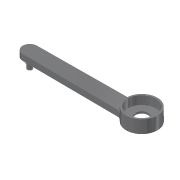
# Autodesk Inventor part: bras_moteur_1
Saved by Autodesk Inventor 2020 (Build 240168000, 168)
## iProperties
Created: 2004-05-22
Part Number: bras_moteur_1
Material: Aluminum-6061
Document SubType Name: Modélisation
Designer: françois CHAILLOT
Density: 2.71 g/cm^3
Appearance: Metal-AL-6061 (Machined)
Control State: 0
Master: False
Checked Out: False
Shininess: 66.0
Length Units: 11269
Angle Units: 11279
Time Units: 11290
Mass Units: 11283
Length Display Precision: 3
Angle Display Precision: 2
Density: 0.0
Volumn: 0.0
Area: 0.0
PropertySet Name: Model Information
Author: françois CHAILLOT
Autodesk Inventor part; units mm, degrees
ref_plane "Plan YZ" through (0, 0, 0) normal (1, 0, 0) x (0, 1, 0)
sketch "Esquisse1" plane through (0, 0, 0) normal (0, 0, 1) x (1, 0, 0)
  line L0 (-51.70019, 0) -> (420.10247, 0)
  arc A0 (0, 18) -> (0, -18) centre (0, 0) ccw
  line L1 (246.520562, 20) -> (-0.145984, 17.999408)
  line L2 (246.520562, -20) -> (-0.145984, -17.999408)
  line L3 (244.42737, 15.982892) -> (-0.113543, 13.99954)
  arc A1 (-0.113543, 13.99954) -> (-0.113537, -13.99954) centre (0, 0) ccw
  line L4 (244.427323, -15.982787) -> (-0.113537, -13.99954)
  circle A2 centre (280.0019, 0) radius 35
  circle A3 centre (280.0019, 0) radius 39
  dimension "d67" = 20
  dimension "d79" = 18
  dimension "d80" = 4
  dimension "d190" = 70
  dimension "d191" = 78
  dimension "d192" = 20
  constraints: 10 point on circle, 8 end point, 4 centre point, 4 coincident, 4 tangent, 1 point on line
  measures "d67" distance from line of L0 L2.start
  measures "d79" radius of A0
  measures "d80" distance between parallel lines of L1 L3
  measures "d190" diameter of A2
  measures "d191" diameter of A3
  measures "d192" distance from line of L0 L1.start
extrude "Extrusion7" add sketch "Esquisse1" along normal blind 15 contours A2 L0 A3 | L0 A3 A2 | A3 L3 A1 L0 A0 L1 | L2 A0 L0 A1 L4 A3
sketch "Esquisse7" plane through (0, 0, 15) normal (0, 0, 1) x (1, 0, 0)
  arc A0 (244.42737, 15.982892) -> (244.427323, -15.982787) centre (280.0019, 0) ccw
  line L0 (-0.113543, 13.99954) -> (244.42737, 15.982892)
  line L1 (244.427323, -15.982787) -> (-0.113537, -13.99954)
  arc A1 (-0.113543, 13.99954) -> (-0.113537, -13.99954) centre (0, 0) ccw
  point P0 (280, 0.667235)
extrude "Extrusion9" add sketch "Esquisse7" against normal blind 4
ref_plane "Plan de construction2" through (0, 0, 11) normal (0, 0, -1) x (-1, 0, 0)
sketch "Esquisse13" plane through (0, 0, 11) normal (0, 0, -1) x (-1, 0, 0)
  circle A0 centre (0, 0) radius 17.99
  line L0 (-65, 15) -> (-15, 15)
  line L1 (-15, 15) -> (-15, -15)
  line L2 (-15, -15) -> (-65, -15)
  line L3 (-65, -15) -> (-65, 15)
  line L4 (-65, -15) -> (-15, 15)
  line L5 (-65, -13.250714) -> (-17.915476, 15)
  line L6 (-62.084524, -15) -> (-15, 13.250714)
  line L7 (-65, 15) -> (-15, -15)
  line L8 (-62.084524, 15) -> (-15, -13.250714)
  line L9 (-65, 13.250714) -> (-17.915476, -15)
  line L10 (-137, 15.5) -> (-75, 15.5)
  line L11 (-75, 15.5) -> (-75, -15.5)
  line L12 (-75, -15.5) -> (-137, -15.5)
  line L13 (-137, -15.5) -> (-137, 15.5)
  line L14 (-137, 15.5) -> (-75, -15.5)
  line L15 (-75, 15.5) -> (-137, -15.5)
  line L16 (-133.645898, 15.5) -> (-75, -13.822949)
  line L17 (-78.354102, 15.5) -> (-137, -13.822949)
  line L18 (-75, 13.822949) -> (-133.645898, -15.5)
  line L19 (-137, 13.822949) -> (-78.354102, -15.5)
  line L20 (-75, 15.5) -> (-65, 15)
  line L21 (-65, -15) -> (-75, -15.994192)
  line L22 (-75, -15.994192) -> (-75, -15.5)
  line L23 (-195, 16) -> (-147, 16)
  line L24 (-147, 16) -> (-147, -16)
  line L25 (-147, -16) -> (-195, -16)
  line L26 (-195, -16) -> (-195, 16)
  line L27 (-195, 16) -> (-147, -16)
  line L28 (-147, 16) -> (-195, -16)
  line L29 (-192.295837, 16) -> (-147, -14.197224)
  line L30 (-195, 14.197224) -> (-149.704163, -16)
  line L31 (-149.704163, 16) -> (-195, -14.197224)
  line L32 (-147, 14.197224) -> (-192.295837, -16)
  line L33 (-238, 8) -> (-221, 10)
  line L34 (-221, 10) -> (-221, -10)
  line L35 (-221, -10) -> (-238, -8)
  line L36 (-238, 8) -> (-238, -8)
  line L37 (-217, 10.000093) -> (-205, 10.000093)
  line L38 (-205, 10.000093) -> (-205, -9.999907)
  line L39 (-205, -9.999907) -> (-217, -9.999907)
  line L40 (-217, -9.999907) -> (-217, 10.000093)
  line L41 (-195, -16) -> (-202.511566, -16.060823)
  line L42 (-195, 17.693981) -> (-195, 16)
  line L43 (-195, -16) -> (-195, -16)
  line L44 (-205, 10.000093) -> (-205, 17.174385)
  line L45 (-147, -16) -> (-137, -15.5)
  line L46 (-205, 17.174385) -> (-195, 17.693981)
  line L47 (-244.732469, -15.983444) -> (-244.732469, -15.983444)
  line L48 (-205, 10.000093) -> (-217, 10.000093)
  line L49 (-217, -9.999907) -> (-205, -9.999907)
  line L50 (-205, -9.999907) -> (-205.000086, -16.080973)
  line L51 (-205.000086, -16.080973) -> (-202.511566, -16.060823)
  line L52 (-205, 15.982892) -> (-205, -15.662243)
  line L53 (-147, 16) -> (-137, 15.5)
  arc A1 (-244.427323, -15.982787) -> (-244.42737, 15.982892) centre (-280.0019, 0) ccw
  circle A2 centre (-70, 0) radius 9
  circle A3 centre (-142, 0) radius 9
  circle A4 centre (-200, 0) radius 9
  line L54 (0, -21.588) -> (0, 28.784)
  line L55 (-244.42737, 15.982892) -> (-205, 15.982892)
  line L56 (-205, 15.982892) -> (-205, 10.000093)
  line L57 (-217, 10.000093) -> (-217, -9.999907)
  line L58 (-205, -9.999907) -> (-205, -15.662243)
  point P0 (-75, 15.186054)
  point P1 (-75, -14.19704)
  point P2 (-280, 0.667235)
  dimension "d100" = 35.98
  dimension "d104" = 50
  dimension "d109" = 1.5
  dimension "d110" = 1.5
  dimension "d118" = 1.5
  dimension "d119" = 1.5
  dimension "d128" = 31
  dimension "d131" = 1.5
  dimension "d132" = 3
  dimension "d134" = 10
  dimension "d135" = 62
  dimension "d148" = 32
  dimension "d150" = 48
  dimension "d151" = 10
  dimension "d153" = 1.5
  dimension "d154" = 3
  dimension "d155" = 1.5
  dimension "d156" = 3
  dimension "d157" = 20
  dimension "d159" = 12
  dimension "d160" = 10
  dimension "d161" = 17
  dimension "d162" = 20
  dimension "d167" = 16
  dimension "d194" = 18
  dimension "d195" = 18
  dimension "d196" = 18
  dimension "d197" = 65
  constraints: 116 end point, 25 point on line, 13 parallel, 6 perpendicular, 4 centre point, 4 coincident, 4 horizontal, 2 collinear
  measures "d100" diameter of A0
  measures "d104" distance between parallel lines of L1 L3
  measures "d109" distance between parallel lines of L6 L4
  measures "d110" distance between parallel lines of L5 L4
  measures "d118" distance between parallel lines of L8 L7
  measures "d119" distance between parallel lines of L9 L7
  measures "d128" distance between parallel lines of L12 L10
  measures "d131" distance between parallel lines of L17 L15
  measures "d132" distance between parallel lines of L18 L17
  measures "d134" distance between parallel lines of L3 L11
  measures "d135" distance between parallel lines of L13 L11
  measures "d148" distance between parallel lines of L25 L23
  measures "d150" distance between parallel lines of L24 L26
  measures "d151" distance between parallel lines of L13 L24
  measures "d153" distance between parallel lines of L29 L27
  measures "d154" distance between parallel lines of L30 L29
  measures "d155" distance between parallel lines of L31 L28
  measures "d156" distance between parallel lines of L31 L32
  measures "d157" distance between parallel lines of L39 L37
  measures "d159" distance between parallel lines of L40 L38
  measures "d160" distance between parallel lines of L26 L38
  measures "d161" distance between parallel lines of L34 L36
  measures "d162" distance of L34.end L33.end
  measures "d167" distance of L35.end L33.start
  measures "d194" diameter of A2
  measures "d195" diameter of A3
  measures "d196" diameter of A4
  measures "d197" distance between parallel lines of L54 L3
extrude "Extrusion19" add sketch "Esquisse13" along normal blind 11 contours A0 L54 | L54 A0 L1 | L1 A0 | L6 L8 L4 L1 | L1 L7 L6 L8 | L4 L8 L5 L0 | L6 L7 L4 L8 | L2 L9 L6 L7 | L4 L7 L5 L8 | L6 L9 L4 L7 | L8 L5 L7 L0 | L4 L9 L5 L7 | L6 L2 L4 L9 | L7 L5 L9 L3 | L3 A2 L11 L20 | L4 L3 L5 L9 | L21 L22 L11 A2 L3 | L15 L16 L17 L10 | L11 L18 L16 L15 | A2 L3 | L3 A2 L11 | L16 L18 L14 L15 | L15 L14 L17 L16 | L14 L18 L16 L11 | L12 L19 L18 L14 | L11 A2 | L16 L17 L14 L10 | L15 L19 L17 L14 | L14 L18 L19 L15 | L14 L17 L19 L13 | L13 A3 L24 L53 | L19 L18 L12 L15 | L15 L13 L17 L19 | L28 L29 L31 L23 | L24 L32 L29 L28 | L45 L24 A3 L13 | A3 L13 | L13 A3 L24 | L29 L32 L27 L28 | L28 L27 L31 L29 | L27 L32 L29 L24 | L25 L30 L32 L27 | L24 A3 | L29 L31 L27 L23 | L28 L30 L31 L27 | L27 L32 L30 L28 | L27 L31 L30 L26 | L26 A4 L38 L44 L46 L42 | L30 L32 L25 L28 | L28 L26 L31 L30 | L41 L51 L50 L38 A4 L26 | A4 L26 | L26 A4 L38 | L38 A4
sketch "Esquisse18" plane through (0, 0, 11) normal (0, 0, -1) x (-1, 0, 0)
  line L0 (-205.00008, -15.663029) -> (-244.427323, -15.982787)
  arc A0 (-244.427323, -15.982787) -> (-244.42737, 15.982892) centre (-280.0019, 0) ccw
  arc A1 (-205, 7.483315) -> (-205, -7.483315) centre (-200, 0) ccw
  line L1 (-205, -9.999907) -> (-205, -7.483315)
  line L2 (-205.00008, -15.663029) -> (-205, -9.999907)
  line L3 (-244.427323, -15.982787) -> (-205.00008, -15.663029)
  line L4 (-205, -9.999907) -> (-217, -9.999907)
  line L5 (-217, -9.999907) -> (-217, 10.000093)
  line L6 (-238, 8) -> (-221, 10)
  line L7 (-221, 10) -> (-221, -10)
  line L8 (-238, 8) -> (-238, -8)
  line L9 (-221, -10) -> (-238, -8)
  line L10 (-65, -7.483315) -> (-65, -13.250714)
  line L11 (-244.42737, 15.982892) -> (-204, 15.982892)
  line L12 (-204, 15.982892) -> (-205, 10.000093)
  line L13 (-65, 13.250714) -> (-65, 7.483315)
  line L14 (-205, 10.000093) -> (-217, 10.000093)
  constraints: 6 end point, 2 perpendicular
extrude "Extrusion20" add sketch "Esquisse18" along normal blind 11
sketch "Esquisse20" plane through (0, 0, 15) normal (0, 0, 1) x (1, 0, 0)
  circle A0 centre (280.0019, 0) radius 35 projected
  circle A1 centre (280.0019, 0) radius 39
  dimension "d202" = 78
  constraints: 1 centre point, 1 coincident
  measures "d202" diameter of A1
extrude "Extrusion21" add sketch "Esquisse20" along normal blind 17
ref_plane "Plan de construction3" through (280.0019, 0, 11) normal (0, 0, 1) x (1, 0, 0)
sketch "Esquisse21" plane through (280.0019, 0, 11) normal (0, 0, 1) x (1, 0, 0)
  circle A0 centre (0, 0) radius 35 projected
  circle A1 centre (35, 0) radius 2
  circle A2 centre (0, 0) radius 15.5
  dimension "d206" = 4
  dimension "d214" = 31
  constraints: 2 centre point, 2 coincident, 1 horizontal alignment, 1 other
  measures "d206" diameter of A1
  measures "d214" diameter of A2
extrude "Extrusion22" add sketch "Esquisse21" along normal blind 21 contours A0 A1 | A0 A1 picked at (34.372994, -0.454527) picked at (35.596147, -0.516389)
pattern_circular "Réseau circulaire1" count 3 over 360 about axis through (280.0019, 0, 0) along (0, 0, 1) of "Extrusion22"
extrude "Extrusion23" add sketch "Esquisse21" against normal blind 5 contours A0 A1 | A1 A0 picked at (34.372994, -0.454527) picked at (27.295087, -4.99456)
sketch "Esquisse22" plane through (0, 0, 0) normal (0, 0, -1) x (-1, 0, 0)
  arc A0 (0.145984, -17.999408) -> (0.145984, 17.999408) centre (0, 0) ccw
  line L0 (0, 9.814955) -> (8.5, 4.907477)
  line L1 (8.5, 4.907477) -> (8.5, -4.907477)
  line L2 (8.5, -4.907477) -> (0, -9.814955)
  line L3 (0, -9.814955) -> (-8.5, -4.907477)
  line L4 (-8.5, -4.907477) -> (-8.5, 4.907477)
  line L5 (-8.5, 4.907477) -> (0, 9.814955)
  circle A1 centre (0, 0) radius 6
  dimension "d215" = 17
  dimension "d216" = 12
  constraints: 12 end point, 2 coincident, 1 centre point, 11 other
  measures "d215" distance between parallel lines of L1 L4
  measures "d216" diameter of A1
extrude "Extrusion24" add sketch "Esquisse22" along normal blind 25.5 contours A1
extrude "Extrusion25" add sketch "Esquisse22" along normal blind 10
ref_plane "Plan de construction4" through (0, 0, -22.5) normal (0, 0, -1) x (-1, 0, 0)
sketch "Esquisse23" plane through (0, 0, -22.5) normal (0, 0, -1) x (-1, 0, 0)
  circle A0 centre (0, 0) radius 6 projected
  circle A1 centre (0, 0) radius 5
  dimension "d222" = 10
  constraints: 1 centre point, 1 coincident
  measures "d222" diameter of A1
extrude "Extrusion26" cut sketch "Esquisse23" along normal blind 1.2
fillet "Congé12" radius 3 2 edges at (15, -14.1221, 5.5) (15, 14.1221, 5.5)
fillet "Congé13" radius 1 2 edges at (11.1839, -14.0912, 5.5) (11.1839, 14.0912, 5.5)
fillet "Congé13" radius 1 51 edges at (42.9155, 0, 5.5) (37.0845, 0, 5.5) (61.2465, -14.4972, 5.5) (61.2465, 14.4972, 5.5) (65, -7.4833, 5.5) (65, 7.4833, 5.5) (40, -1.7493, 5.5) (40, 1.7493, 5.5) (65, -13.2507, 5.5) (65, 13.2507, 5.5) (106, -1.6771, 5.5) (132.8009, -15.0775, 5.5) (102.6459, 0, 5.5) (75, -13.8229, 5.5) (75, 7.4833, 5.5) (80.0546, 14.6497, 5.5) (75, -7.4833, 5.5) (75, 13.8229, 5.5) (106, 1.6771, 5.5) (80.0547, -14.6497, 5.5) (137, -13.8229, 5.5) (137, 7.4833, 5.5) (109.3541, 0, 5.5) (147, -7.4833, 5.5) (173.7042, 0, 5.5) (150.868, 15.2241, 5.5) (147, 7.4833, 5.5) (132.801, 15.0775, 5.5) (137, 13.8229, 5.5) (171, -1.8028, 5.5) (168.2958, 0, 5.5) (171, 1.8028, 5.5) (150.8681, -15.224, 5.5) (147, 14.1972, 5.5) (147, -14.1972, 5.5) (195, 14.1972, 5.5) (195, -7.4833, 5.5) (191.6278, 15.5547, 5.5) (217, 10.0001, 5.5) (221, 10, 5.5) (205, 10.0001, 5.5) (205, -9.9999, 5.5) (217, -9.9999, 5.5) (195, -14.1972, 5.5) (191.6277, -15.5546, 5.5) (195, 7.4833, 5.5) (238, 8, 5.5) (238, -8, 5.5) (221, -10, 5.5) (205, 7.4833, 5.5) (205, -7.4833, 5.5)
sketch "Esquisse24" plane through (0, 0, 0) normal (0, 0, -1) x (-1, 0, 0)
  arc A0 (-191, 0) -> (-194.6, 7.2) centre (-200, 0) ccw projected
  arc A1 (-75.4, 7.2) -> (-75.4, -7.2) centre (-70, 0) ccw projected
  arc A2 (-133, 0) -> (-136.6, 7.2) centre (-142, 0) ccw projected
  constraints: 3 coincident
hole "Perçage6" at (70, 0, 0) at (142, 0, 0) at (200, 0, 0) direction (0, 0, 1) diameter 3 depth 2.58 tip angle 90 countersink diameter 8 countersink angle 90
fillet "Congé14" radius 15 2 edges at (246.5206, -20, 7.5) (246.5206, 20, 7.5)
